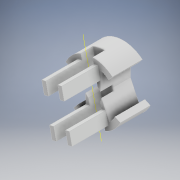
# Autodesk Inventor part: Spinner
Saved by Autodesk Inventor 2020 (Build 240168000, 168)
## iProperties
Created: 2019-12-02
Part Number: Spinner
Material: 일반
Document SubType Name: Modeling
Designer: Knowblesse
Density: 1 g/cm^3
Appearance: 기본값
Author: Knowblesse
## iProperties of the stored document _3D 인쇄.ipt
Created: 2019-12-02
Part Number: _3D 인쇄
Material: 일반
Document SubType Name: Modeling
Designer: Knowblesse
Density: 1 g/cm^3
Appearance: 기본값
Author: Knowblesse
Autodesk Inventor part; units mm, degrees
ref_plane "YZ Plane" through (0, 0, 0) normal (1, 0, 0) x (0, 1, 0)
ref_plane "XZ Plane" through (0, 0, 0) normal (0, 1, 0) x (-1, 0, 0)
ref_plane "XY Plane" through (0, 0, 0) normal (0, 0, 1) x (1, 0, 0)
sketch "스케치2" plane through (0, 0, 0) normal (0, 0, 1) x (1, 0, 0)
  circle A0 centre (0, 0) radius 9
  line L0 (-3.05, -9.5235) -> (-3.05, -0.6762)
  line L1 (-3.05, -0.6762) -> (-6.7891, 7.3423)
  line L2 (3.05, 9.5235) -> (3.05, 0.6762)
  line L3 (3.05, 0.6762) -> (7.8873, -9.6974)
  line L4 (-3.05, -0.6762) -> (3.05, 0.6762) construction
  circle A1 centre (0, 0) radius 12.5
  line L5 (-11.3288, 5.2827) -> (11.3288, -5.2827)
  line L6 (8.0348, 9.5756) -> (-8.0348, -9.5756)
  circle A2 centre (0, 0) radius 10
  point P0 (5.7851, 6.8944)
  point P1 (-8.1568, 3.8036)
  point P2 (6.3427, -6.3851)
  point P3 (-5.7851, -6.8944)
  point P4 (8.1568, -3.8036)
  point P5 (-6.4279, -7.6604)
  point P6 (9.0631, -4.2262)
  point P7 (6.7891, -7.3423)
  point P8 (6.4279, 7.6604)
  point P9 (-9.0631, 4.2262)
  dimension "d12" = 18
  dimension "d14" = 6.1
  dimension "d15" = 25
  dimension "d16" = 6.1
  dimension "d17" = 25
  dimension "d19" = 40
  dimension "d20" = 40
  dimension "d36" = 20
  constraints: 14 end point, 8 point on circle, 4 coincident, 3 centre point, 3 midpoint, 2 vertical, 1 parallel
  measures "d12" diameter of A0
  measures "d14" distance between parallel lines of L0 L2
  measures "d15" angle of L1 L0
  measures "d16" distance between parallel lines of L3 L1
  measures "d17" diameter of A1
  measures "d19" angle of L1 L5
  measures "d20" angle of L6 L2
  measures "d36" diameter of A2
extrude "돌출1" add sketch "스케치2" along normal blind 12.5 contours L2 L6 L5 L1 A0 | A0 L1 A2 L2 | A2 L5 A1 L6 | L2 L3 L5 L6 | L3 A2 L0 A0 | A0 L0 L6 L5 L3 | L5 A1 L3 A2 | L6 L0 L1 L5 | L3 A1 L6 A2 picked at (3.8905, 10.9384)
sketch "스케치3" plane through (0, 0, 12.5) normal (0, 0, 1) x (1, 0, 0)
  arc A0 (8.0348, 9.5756) -> (-11.3288, 5.2827) centre (0, 0) ccw projected
  line L0 (-11.3288, 5.2827) -> (-9.0631, 4.2262) projected
  line L1 (-6.7891, 7.3423) -> (-3.05, -0.6762) projected
  line L2 (-3.05, -0.6762) -> (-3.05, -9.5235) projected
  line L3 (-6.4279, -7.6604) -> (-8.0348, -9.5756) projected
  arc A1 (-8.0348, -9.5756) -> (11.3288, -5.2827) centre (0, 0) ccw projected
  line L4 (11.3288, -5.2827) -> (9.0631, -4.2262) projected
  line L5 (6.7891, -7.3423) -> (3.05, 0.6762) projected
  line L6 (3.05, 0.6762) -> (3.05, 9.5235) projected
  line L7 (6.4279, 7.6604) -> (8.0348, 9.5756) projected
  arc A2 (8.0348, 9.5756) -> (-11.3288, 5.2827) centre (0, 0) ccw projected
  line L8 (-2.7055, 12.2037) -> (2.7055, -12.2037)
  arc A3 (-8.0348, -9.5756) -> (11.3288, -5.2827) centre (0, 0) ccw projected
  line L9 (3.05, 0.6762) -> (3.05, 9.5235) projected
  line L10 (-3.05, -0.6762) -> (3.05, 0.6762)
  line L11 (-3.5229, 4.3404) -> (-4.6051, 9.2219)
  line L12 (-4.6051, 9.2219) -> (-6.2966, 8.8469)
  line L13 (-6.2966, 8.8469) -> (-5.2144, 3.9654)
  line L14 (-5.2144, 3.9654) -> (-3.5229, 4.3404)
  line L15 (-3.5229, 4.3404) -> (-6.2966, 8.8469) construction
  line L16 (-4.6051, 9.2219) -> (-5.2144, 3.9654) construction
  line L17 (1.3585, 5.4226) -> (0.2763, 10.3041)
  line L18 (0.2763, 10.3041) -> (1.9678, 10.679)
  line L19 (1.9678, 10.679) -> (3.05, 5.7976)
  line L20 (3.05, 5.7976) -> (1.3585, 5.4226)
  line L21 (1.3585, 5.4226) -> (1.9678, 10.679) construction
  line L22 (0.2763, 10.3041) -> (3.05, 5.7976) construction
  line L23 (-1.3585, -5.4226) -> (-0.2763, -10.3041)
  line L24 (-0.2763, -10.3041) -> (-1.9678, -10.679)
  line L25 (-1.9678, -10.679) -> (-3.05, -5.7976)
  line L26 (-3.05, -5.7976) -> (-1.3585, -5.4226)
  line L27 (-1.3585, -5.4226) -> (-1.9678, -10.679) construction
  line L28 (-0.2763, -10.3041) -> (-3.05, -5.7976) construction
  line L29 (3.5229, -4.3404) -> (4.6051, -9.2219)
  line L30 (4.6051, -9.2219) -> (5.2144, -3.9654) construction
  line L31 (4.6051, -9.2219) -> (6.2966, -8.8469)
  line L32 (6.2966, -8.8469) -> (5.2144, -3.9654)
  line L33 (5.2144, -3.9654) -> (3.5229, -4.3404)
  line L34 (3.5229, -4.3404) -> (6.2966, -8.8469) construction
  arc A4 (-6.7891, 7.3423) -> (-9.0631, 4.2262) centre (0, 0) ccw projected
  arc A5 (-6.4279, -7.6604) -> (-3.05, -9.5235) centre (0, 0) ccw projected
  arc A6 (6.7891, -7.3423) -> (9.0631, -4.2262) centre (0, 0) ccw projected
  arc A7 (6.4279, 7.6604) -> (3.05, 9.5235) centre (0, 0) ccw projected
  point P0 (3.05, 8.4674)
  point P1 (-4.9098, 6.5936)
  point P2 (1.6632, 8.0508)
  point P3 (-1.6632, -8.0508)
  point P4 (4.9098, -6.5936)
  dimension "d32" = 2.5
  dimension "d33" = 5
  dimension "d35" = 5
  constraints: 52 end point, 15 symmetric about line, 8 midpoint, 4 point on circle, 3 parallel, 1 perpendicular, 1 point on line
  measures "d32" distance between parallel lines of L8 L11
  measures "d33" distance between parallel lines of L12 L14
  measures "d35" distance between parallel lines of L10 L14
extrude "돌출2" add sketch "스케치3" along normal blind 15 contours L20 L17 L18 L19 | L13 L12 L11 L14 | L32 L31 L29 L33 | L26 L23 L24 L25
sketch "스케치4" plane through (0, 0, 12.5) normal (0, 0, 1) x (1, 0, 0)
  line L0 (0.2648, -12.7448) -> (-5.1462, 11.6626)
  line L1 (-5.1462, 11.6626) -> (-0.2648, 12.7448)
  line L2 (-0.2648, 12.7448) -> (5.1462, -11.6626)
  line L3 (5.1462, -11.6626) -> (0.2648, -12.7448)
  line L4 (0.2648, -12.7448) -> (-0.2648, 12.7448) construction
  line L5 (-5.1462, 11.6626) -> (5.1462, -11.6626) construction
  line L6 (-5.0577, 22.8136) -> (5.0577, -22.8136) projected
  circle A0 centre (0, 0) radius 3.5
  line L7 (-6.4279, -7.6604) -> (-8.0348, -9.5756) projected
  arc A1 (-8.0348, -9.5756) -> (11.3288, -5.2827) centre (0, 0) ccw projected
  line L8 (11.3288, -5.2827) -> (9.0631, -4.2262) projected
  arc A2 (6.7891, -7.3423) -> (9.0631, -4.2262) centre (0, 0) ccw projected
  line L9 (6.7891, -7.3423) -> (5.2144, -3.9654) projected
  line L10 (5.2144, -3.9654) -> (6.2966, -8.8469) projected
  line L11 (6.2966, -8.8469) -> (4.6051, -9.2219) projected
  line L12 (4.6051, -9.2219) -> (3.5229, -4.3404) projected
  line L13 (3.5229, -4.3404) -> (5.2144, -3.9654) projected
  line L14 (5.2144, -3.9654) -> (3.05, 0.6762) projected
  line L15 (3.05, 0.6762) -> (3.05, 5.7976) projected
  line L16 (3.05, 5.7976) -> (1.3585, 5.4226) projected
  line L17 (1.3585, 5.4226) -> (0.2763, 10.3041) projected
  line L18 (0.2763, 10.3041) -> (1.9678, 10.679) projected
  line L19 (1.9678, 10.679) -> (3.05, 5.7976) projected
  line L20 (3.05, 5.7976) -> (3.05, 9.5235) projected
  arc A3 (6.4279, 7.6604) -> (3.05, 9.5235) centre (0, 0) ccw projected
  line L21 (6.4279, 7.6604) -> (8.0348, 9.5756) projected
  arc A4 (8.0348, 9.5756) -> (-11.3288, 5.2827) centre (0, 0) ccw projected
  line L22 (-11.3288, 5.2827) -> (-9.0631, 4.2262) projected
  arc A5 (-6.7891, 7.3423) -> (-9.0631, 4.2262) centre (0, 0) ccw projected
  line L23 (-6.7891, 7.3423) -> (-5.2144, 3.9654) projected
  line L24 (-5.2144, 3.9654) -> (-6.2966, 8.8469) projected
  line L25 (-6.2966, 8.8469) -> (-4.6051, 9.2219) projected
  line L26 (-4.6051, 9.2219) -> (-3.5229, 4.3404) projected
  line L27 (-3.5229, 4.3404) -> (-5.2144, 3.9654) projected
  line L28 (-5.2144, 3.9654) -> (-3.05, -0.6762) projected
  line L29 (-3.05, -0.6762) -> (-3.05, -5.7976) projected
  line L30 (-3.05, -5.7976) -> (-1.3585, -5.4226) projected
  line L31 (-1.3585, -5.4226) -> (-0.2763, -10.3041) projected
  line L32 (-0.2763, -10.3041) -> (-1.9678, -10.679) projected
  line L33 (-1.9678, -10.679) -> (-3.05, -5.7976) projected
  line L34 (-3.05, -5.7976) -> (-3.05, -9.5235) projected
  arc A6 (-6.4279, -7.6604) -> (-3.05, -9.5235) centre (0, 0) ccw projected
  line L35 (-1.3585, -5.4226) -> (-3.05, -5.7976) projected
  line L36 (-3.05, -5.7976) -> (-1.9678, -10.679) projected
  line L37 (-1.9678, -10.679) -> (-0.2763, -10.3041) projected
  line L38 (-0.2763, -10.3041) -> (-1.3585, -5.4226) projected
  line L39 (6.2966, -8.8469) -> (5.2144, -3.9654) projected
  line L40 (5.2144, -3.9654) -> (3.5229, -4.3404) projected
  line L41 (3.5229, -4.3404) -> (4.6051, -9.2219) projected
  line L42 (4.6051, -9.2219) -> (6.2966, -8.8469) projected
  point P0 (1.9106, 2.9325)
  point P1 (2.9709, -1.8503)
  point P2 (-2.9709, 1.8503)
  point P3 (-1.9106, -2.9325)
  dimension "d37" = 7
  constraints: 12 end point, 3 parallel, 2 midpoint, 1 centre point, 1 coincident, 1 perpendicular, 1 point on line, 1 tangent
  measures "d37" diameter of A0
extrude "돌출3" cut sketch "스케치4" against normal blind 5 contours L0 A0 L6 A1 | A1 L3 L0 | A0 L29 L28 L0 | L0 A0 L6 | A1 L2 L3 | L6 A0 L2 A1 | L0 A4 L6 A0 | A0 L28 L29 | L6 A0 L2 | L6 A4 L2 A0 | L2 A0 L15 L14 | A4 L0 L1 | L1 L2 A4 | L14 L15 A0
